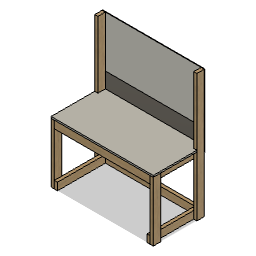
workdesk_v1 (Autodesk Fusion 360 design; units mm, degrees)
Autodesk Fusion 360 part; units mm, degrees
sketch "Sketch1" plane through (0, 0, 0) normal (0, 1, 0) x (1, 0, 0)
  line L0 (0, 0) -> (38.1, 0)
  line L1 (38.1, 0) -> (38.1, 88.9)
  line L2 (38.1, 88.9) -> (0, 88.9)
  line L3 (0, 88.9) -> (0, 0)
  line L4 (1181.1, 88.9) -> (1181.1, 0)
  line L5 (1219.2, 88.9) -> (1181.1, 88.9)
  line L6 (1219.2, 0) -> (1219.2, 88.9)
  line L7 (1181.1, 0) -> (1219.2, 0)
  line L8 (38.1, 609.6) -> (0, 609.6)
  line L9 (0, 609.6) -> (0, 520.7)
  line L10 (0, 520.7) -> (38.1, 520.7)
  line L11 (38.1, 520.7) -> (38.1, 609.6)
  line L12 (1219.2, 609.6) -> (1181.1, 609.6)
  line L13 (1181.1, 609.6) -> (1181.1, 520.7)
  line L14 (1219.2, 520.7) -> (1219.2, 609.6)
  line L15 (1181.1, 520.7) -> (1219.2, 520.7)
  dimension "d7" = 38.1
  dimension "d8" = 88.9
  dimension "d9" = 38.1
  dimension "d10" = 88.9
  dimension "d11" = 38.1
  dimension "d12" = 88.9
  dimension "d13" = 38.1
  dimension "d14" = 88.9
  constraint horizontal L0
  constraint vertical L1
  constraint horizontal L2
  constraint vertical L3
  constraint coincident L0.start L3.end
  constraint horizontal L7
  constraint vertical L6
  constraint horizontal L5
  constraint vertical L4
  constraint horizontal L10
  constraint vertical L11
  constraint horizontal L8
  constraint vertical L9
  constraint horizontal L15
  constraint vertical L14
  constraint horizontal L12
  constraint vertical L13
  measures "d7" distance of L0.start L0.end
  measures "d8" distance of L0.start L2.end
  measures "d9" distance of L6.start L4.end
  measures "d10" distance of L4.start L4.end
  measures "d11" distance of L10.end L9.end
  measures "d12" distance of L8.end L9.end
  measures "d13" distance of L13.end L14.start
  measures "d14" distance of L13.end L12.end
extrude "Extrude1" add sketch "Sketch1" along normal blind 711.2 contours L0 L1 L2 L3 | L4 L5 L6 L7 makes body 1 at (0, 237.0667, -59.2667) makes body 2 at (1219.2, 237.0667, -29.6333)
extrude "Extrude2" add sketch "Sketch1" along normal blind 1339.85 separate body contours L8 L9 L10 L11 | L12 L13 L14 L15 makes body 3 at (38.1, 893.2333, -550.3333) makes body 4 at (1219.2, 893.2333, -550.3333)
sketch "Sketch3" plane through (38.1, 0, 0) normal (1, 0, 0) x (0, 0, -1)
  line L0 (0, 0) -> (88.9, 0)
  line L1 (88.9, 0) -> (88.9, 711.2)
  line L2 (88.9, 711.2) -> (0, 711.2)
  line L3 (0, 711.2) -> (0, 0)
  line L4 (0, 711.2) -> (38.1, 711.2)
  line L5 (38.1, 711.2) -> (38.1, 622.3)
  line L6 (38.1, 622.3) -> (0, 622.3)
  line L7 (0, 622.3) -> (0, 711.2)
  line L8 (609.6, 711.2) -> (609.6, 622.3)
  line L9 (571.5, 711.2) -> (609.6, 711.2)
  line L10 (571.5, 622.3) -> (571.5, 711.2)
  line L11 (609.6, 622.3) -> (571.5, 622.3)
  dimension "d25" = 38.1
  dimension "d26" = 88.9
  dimension "d27" = 38.1
  dimension "d28" = 88.9
  constraint horizontal L4
  constraint vertical L5
  constraint horizontal L6
  constraint vertical L7
  constraint coincident L2.end L3.start
  constraint horizontal L9
  constraint vertical L8
  constraint horizontal L11
  constraint vertical L10
  measures "d25" distance of L2.end L4.end
  measures "d26" distance of L2.end L6.end
  measures "d27" distance of L9.start L8.start
  measures "d28" distance of L9.start L10.start
extrude "Extrude4" add sketch "Sketch3" along normal blind 1143 separate body contours L2 L3 L4 L5 L6 L7 | L8 L9 L10 L11 makes body 5 at (419.1, 681.5667, -609.6) makes body 6 at (419.1, 681.5667, 0)
sketch "Sketch4" plane through (0, 0, -571.5) normal (0, 0, 1) x (1, 0, 0)
  line L0 (38.1, 711.2) -> (38.1, 622.3)
  line L1 (38.1, 622.3) -> (1181.1, 622.3)
  line L2 (1181.1, 622.3) -> (1181.1, 711.2)
  line L3 (1181.1, 711.2) -> (38.1, 711.2)
  line L4 (38.1, 711.2) -> (76.2, 711.2)
  line L5 (76.2, 711.2) -> (76.2, 622.3)
  line L6 (76.2, 622.3) -> (38.1, 622.3)
  line L7 (38.1, 622.3) -> (38.1, 711.2)
  line L8 (1143, 711.2) -> (1181.1, 711.2)
  line L9 (1143, 622.3) -> (1143, 711.2)
  line L10 (1181.1, 711.2) -> (1181.1, 622.3)
  line L11 (1181.1, 622.3) -> (1143, 622.3)
  line L12 (628.65, 711.2) -> (628.65, 622.3)
  line L13 (590.55, 622.3) -> (590.55, 711.2)
  line L14 (590.55, 711.2) -> (628.65, 711.2)
  line L15 (628.65, 622.3) -> (590.55, 622.3)
  dimension "d31" = 38.1
  dimension "d32" = 88.9
  dimension "d33" = 38.1
  dimension "d34" = 88.9
  dimension "d35" = 38.1
  dimension "d36" = 88.9
  constraint horizontal L4
  constraint vertical L5
  constraint horizontal L6
  constraint vertical L7
  constraint coincident L0.start L3.end
  constraint horizontal L8
  constraint vertical L10
  constraint horizontal L11
  constraint vertical L9
  constraint horizontal L14
  constraint vertical L12
  constraint horizontal L15
  constraint vertical L13
  measures "d31" distance of L0.start L4.end
  measures "d32" distance of L0.start L0.end
  measures "d33" distance of L2.end L8.start
  measures "d34" distance of L8.start L9.start
  measures "d35" distance of L12.start L13.end
  measures "d36" distance of L13.end L13.start
extrude "Extrude5" add sketch "Sketch4" along normal blind 533.4 separate body contours L0 L1 L3 L4 L5 L6 L7 | L1 L3 L12 L13 L14 L15 | L1 L2 L3 L8 L9 L10 L11 makes body 7 at (76.2, 681.5667, -393.7) makes body 8 at (628.65, 681.5667, -393.7) makes body 9 at (1181.1, 651.9333, -393.7)
copy_body "CopyPasteBodies1" bodies 9 7 5 makes body 10 makes body 11 makes body 12
move_body "Move1" bodies 10 11 12 to x (1, 0, 0) y (0, 1, 0) z (0, 0, 1) at (0, -622.3, 0)
move_face "OffsetFaces1" offset 38.1 2 faces at (63.5, 29.6333, -38.1) (1155.7, 59.2667, -38.1) on bodies 10 11
sketch "Sketch5" plane through (0, 711.2, 0) normal (0, 1, 0) x (-1, 0, 0)
  line L0 (0, -88.9) -> (0, 0)
  line L1 (0, 0) -> (-38.1, 0)
  line L2 (-38.1, 0) -> (-38.1, -88.9)
  line L3 (-38.1, -88.9) -> (0, -88.9)
  line L4 (0, 0) -> (-1219.2, 0)
  line L5 (-1219.2, 0) -> (-1219.2, -609.6)
  line L6 (-1219.2, -609.6) -> (0, -609.6)
  line L7 (0, -609.6) -> (0, 0)
  line L8 (0, -609.6) -> (-38.1, -609.6)
  line L9 (-38.1, -609.6) -> (-38.1, -520.7)
  line L10 (-38.1, -520.7) -> (0, -520.7)
  line L11 (0, -520.7) -> (0, -609.6)
  line L12 (-1219.2, -609.6) -> (-1181.1, -609.6)
  line L13 (-1181.1, -609.6) -> (-1181.1, -520.7)
  line L14 (-1181.1, -520.7) -> (-1219.2, -520.7)
  line L15 (-1219.2, -520.7) -> (-1219.2, -609.6)
  dimension "d41" = 1219.2
  dimension "d42" = 609.6
  dimension "d43" = 38.1
  dimension "d44" = 88.9
  dimension "d45" = 38.1
  dimension "d46" = 88.9
  constraint horizontal L4
  constraint vertical L5
  constraint horizontal L6
  constraint vertical L7
  constraint coincident L0.end L1.start
  constraint horizontal L8
  constraint vertical L9
  constraint horizontal L10
  constraint vertical L11
  constraint horizontal L12
  constraint vertical L13
  constraint horizontal L14
  constraint vertical L15
  measures "d41" distance of L0.end L4.end
  measures "d42" distance of L0.end L6.end
  measures "d43" distance of L6.end L8.end
  measures "d44" distance of L6.end L10.end
  measures "d45" distance of L5.end L12.end
  measures "d46" distance of L5.end L14.end
extrude "Extrude6" add sketch "Sketch5" along normal blind 19.05 separate body contours L0 L1 L2 L3 L4 L7 | L2 L3 L4 L5 L6 L7 L9 L10 L13 L14 makes body 13
sketch "Sketch6" plane through (0, 0, -609.6) normal (0, 0, -1) x (-1, 0, 0)
  line L0 (-38.1, 0) -> (0, 0)
  line L1 (0, 0) -> (0, 1339.85)
  line L2 (0, 1339.85) -> (-38.1, 1339.85)
  line L3 (-38.1, 1339.85) -> (-38.1, 0)
  line L4 (0, 1339.85) -> (-1219.2, 1339.85)
  line L5 (-1219.2, 1339.85) -> (-1219.2, 730.25)
  line L6 (-1219.2, 730.25) -> (0, 730.25)
  line L7 (0, 730.25) -> (0, 1339.85)
  dimension "d49" = 1219.2
  dimension "d50" = 609.6
  constraint horizontal L4
  constraint vertical L5
  constraint horizontal L6
  constraint vertical L7
  constraint coincident L1.end L2.start
  measures "d49" distance of L1.end L4.end
  measures "d50" distance of L1.end L6.end
extrude "Extrude7" add sketch "Sketch6" along normal blind 6.35 separate body contours L3 L4 L5 L6 | L1 L2 L3 L4 L6 L7 makes body 14
move_face "OffsetFaces2" offset 184.15 2 faces at (1206.5, 1339.85, -550.3333) (25.4, 1339.85, -550.3333) on bodies 3 4
move_body "Move2" bodies 14 to x (1, 0, 0) y (0, 1, 0) z (0, 0, 1) at (0, 184.15, 0)
sketch "Sketch7" plane through (0, 0, -609.6) normal (0, 0, -1) x (-1, 0, 0)
  line L0 (-38.1, 0) -> (0, 0)
  line L1 (0, 0) -> (0, 1524)
  line L2 (0, 1524) -> (-38.1, 1524)
  line L3 (-38.1, 1524) -> (-38.1, 0)
  line L4 (0, 914.4) -> (-1219.2, 914.4)
  line L5 (-1219.2, 914.4) -> (-1219.2, 660.4)
  line L6 (-1219.2, 660.4) -> (0, 660.4)
  line L7 (0, 660.4) -> (0, 914.4)
  constraint horizontal L4
  constraint vertical L5
  constraint horizontal L6
  constraint vertical L7
  constraint coincident L1 L4.start
extrude "Extrude8" add sketch "Sketch7" along normal blind 6.35 separate body contours L3 L4 L5 L6 | L1 L3 L4 L6 L7 makes body 15
equation "bench_height = 28 in"
equation "top_thickness = 0.75 in"
equation "wood_width = 1.5 in"
equation "wood_height = 3.5 in"
equation "top_length = 4 ft"
equation "top_depth = 2 ft"
equation "d7 = wood_width"
equation "d8 = wood_height"
equation "d9 = wood_width"
equation "d10 = wood_height"
equation "d11 = wood_width"
equation "d12 = wood_height"
equation "d13 = wood_width"
equation "d14 = wood_height"
equation "d15 = bench_height"
equation "d17 = bench_height + top_thickness + top_depth"
equation "d25 = wood_width"
equation "d26 = wood_height"
equation "d27 = wood_width"
equation "d28 = wood_height"
equation "d29 = top_length - wood_width * 2"
equation "d31 = wood_width"
equation "d32 = wood_height"
equation "d33 = wood_width"
equation "d34 = wood_height"
equation "d35 = wood_width"
equation "d36 = wood_height"
equation "d37 = top_depth - wood_width * 2"
equation "d39 = wood_width"
equation "pegboard_thickness = 0.25 in"
equation "d41 = top_length"
equation "d42 = top_depth"
equation "d43 = wood_width"
equation "d44 = wood_height"
equation "d45 = wood_width"
equation "d46 = wood_height"
equation "d47 = top_thickness"
equation "d49 = top_length"
equation "d50 = top_depth"
equation "d51 = pegboard_thickness"
equation "d54 = pegboard_thickness"
named bodies: "Front Leg (1)", "Front Leg (2)", "Rear Leg (1)", "Rear Leg (2)", "Cross Support (1)", "Cross Support (3)", "Top Depth Support (1)", "Top Depth Support (2)", "Top Depth Support (3)", "Bottom Depth Support (1)", "Bottom Depth Support (2)", "Cross Support (2)", "TableTop", "Pegboard"
